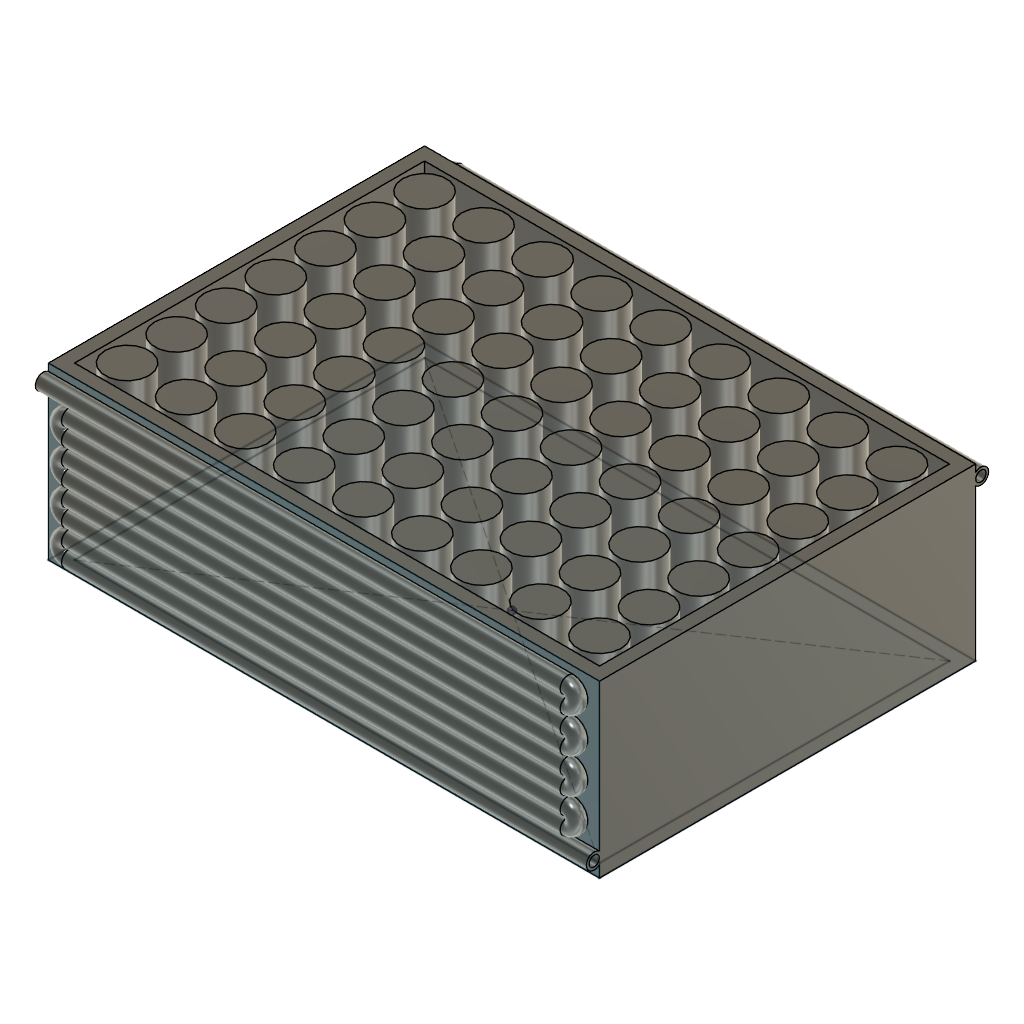
BATTERY_PACK_11 (Autodesk Fusion 360 design; units mm, degrees)
Autodesk Fusion 360 part; units mm, degrees
sketch "Sketch1" plane through (0, 0, 0) normal (0, 0, 1) x (1, 0, 0)
  line L0 (150, 100) -> (-150, 100)
  line L1 (-150, 100) -> (-150, -100)
  line L2 (-150, -100) -> (150, -100)
  line L3 (150, -100) -> (150, 100)
  line L4 (150, 100) -> (-150, -100) construction
  line L5 (-150, 100) -> (150, -100) construction
  line L6 (-157.5, -107.5) -> (157.5, -107.5)
  line L7 (157.5, -107.5) -> (157.5, 107.5)
  line L8 (157.5, 107.5) -> (-157.5, 107.5)
  line L9 (-157.5, 107.5) -> (-157.5, -107.5)
  dimension "d1" = 300
  dimension "d2" = 200
  dimension "d3" = 7.5
  constraint horizontal L0
  constraint perpendicular L0 L1
  constraint parallel L0 L2
  constraint parallel L1 L3
  constraint coincident L4 origin
  constraint coincident L5 origin
  measures "d1" distance of L1.end L2.end
  measures "d2" distance of L0.end L1.end
extrude "Extrude1" add sketch "Sketch1" along normal blind 7.5 contours L0 L1 L2 L3
extrude "Extrude2" add sketch "Sketch1" along normal blind 97.5
sketch "Sketch2" plane through (0, 0, 7.5) normal (0, 0, 1) x (-1, 0, 0)
  line L0 (-150, 100) -> (-150, -100)
  line L1 (-150, -100) -> (150, -100)
  line L2 (150, -100) -> (150, 100)
  line L3 (150, 100) -> (-150, 100)
  circle A0 centre (0, 0) radius 12.5
  circle A1 centre (33.75, 0) radius 12.5
  circle A2 centre (67.5, 0) radius 12.5
  circle A3 centre (101.25, 0) radius 12.5
  circle A4 centre (135, 0) radius 12.5
  circle A5 centre (0, 28.3333) radius 12.5
  circle A6 centre (33.75, 28.3333) radius 12.5
  circle A7 centre (67.5, 28.3333) radius 12.5
  circle A8 centre (101.25, 28.3333) radius 12.5
  circle A9 centre (135, 28.3333) radius 12.5
  circle A10 centre (0, 56.6667) radius 12.5
  circle A11 centre (33.75, 56.6667) radius 12.5
  circle A12 centre (67.5, 56.6667) radius 12.5
  circle A13 centre (101.25, 56.6667) radius 12.5
  circle A14 centre (135, 56.6667) radius 12.5
  circle A15 centre (0, 85) radius 12.5
  circle A16 centre (33.75, 85) radius 12.5
  circle A17 centre (67.5, 85) radius 12.5
  circle A18 centre (101.25, 85) radius 12.5
  circle A19 centre (135, 85) radius 12.5
  circle A20 centre (33.75, 0) radius 12.5
  circle A21 centre (67.5, 0) radius 12.5
  circle A22 centre (101.25, 0) radius 12.5
  circle A23 centre (135, 0) radius 12.5
  circle A24 centre (0, -28.3333) radius 12.5
  circle A25 centre (33.75, -28.3333) radius 12.5
  circle A26 centre (67.5, -28.3333) radius 12.5
  circle A27 centre (101.25, -28.3333) radius 12.5
  circle A28 centre (135, -28.3333) radius 12.5
  circle A29 centre (0, -56.6667) radius 12.5
  circle A30 centre (33.75, -56.6667) radius 12.5
  circle A31 centre (67.5, -56.6667) radius 12.5
  circle A32 centre (101.25, -56.6667) radius 12.5
  circle A33 centre (135, -56.6667) radius 12.5
  circle A34 centre (0, -85) radius 12.5
  circle A35 centre (33.75, -85) radius 12.5
  circle A36 centre (67.5, -85) radius 12.5
  circle A37 centre (101.25, -85) radius 12.5
  circle A38 centre (135, -85) radius 12.5
  circle A39 centre (-33.75, 0) radius 12.5
  circle A40 centre (-67.5, 0) radius 12.5
  circle A41 centre (-101.25, 0) radius 12.5
  circle A42 centre (-135, 0) radius 12.5
  circle A43 centre (0, -28.3333) radius 12.5
  circle A44 centre (-33.75, -28.3333) radius 12.5
  circle A45 centre (-67.5, -28.3333) radius 12.5
  circle A46 centre (-101.25, -28.3333) radius 12.5
  circle A47 centre (-135, -28.3333) radius 12.5
  circle A48 centre (0, -56.6667) radius 12.5
  circle A49 centre (-33.75, -56.6667) radius 12.5
  circle A50 centre (-67.5, -56.6667) radius 12.5
  circle A51 centre (-101.25, -56.6667) radius 12.5
  circle A52 centre (-135, -56.6667) radius 12.5
  circle A53 centre (0, -85) radius 12.5
  circle A54 centre (-33.75, -85) radius 12.5
  circle A55 centre (-67.5, -85) radius 12.5
  circle A56 centre (-101.25, -85) radius 12.5
  circle A57 centre (-135, -85) radius 12.5
  circle A58 centre (-33.75, 0) radius 12.5
  circle A59 centre (-67.5, 0) radius 12.5
  circle A60 centre (-101.25, 0) radius 12.5
  circle A61 centre (-135, 0) radius 12.5
  circle A62 centre (0, 28.3333) radius 12.5
  circle A63 centre (-33.75, 28.3333) radius 12.5
  circle A64 centre (-67.5, 28.3333) radius 12.5
  circle A65 centre (-101.25, 28.3333) radius 12.5
  circle A66 centre (-135, 28.3333) radius 12.5
  circle A67 centre (0, 56.6667) radius 12.5
  circle A68 centre (-33.75, 56.6667) radius 12.5
  circle A69 centre (-67.5, 56.6667) radius 12.5
  circle A70 centre (-101.25, 56.6667) radius 12.5
  circle A71 centre (-135, 56.6667) radius 12.5
  circle A72 centre (0, 85) radius 12.5
  circle A73 centre (-33.75, 85) radius 12.5
  circle A74 centre (-67.5, 85) radius 12.5
  circle A75 centre (-101.25, 85) radius 12.5
  circle A76 centre (-135, 85) radius 12.5
  dimension "d8" = 25
  dimension "d11" = 135
  dimension "d12" = 85
  dimension "d15" = 135
  dimension "d16" = -85
  dimension "d19" = -135
  dimension "d20" = -85
  dimension "d23" = -135
  dimension "d24" = 85
  constraint coincident A0.centre origin
  measures "d8" diameter of A0
extrude "Extrude3" add sketch "Sketch2" along normal blind 90 contours A0 | A1 A20 | A2 A21 | A3 A22 | A4 A23 | A5 A62 | A6 | A7 | A8 | A9 | A10 A67 | A11 | A12 | A13 | A14 | A15 A72 | A16 | A17 | A18 | A19 | A24 A43 | A25 | A26 | A27 | A28 | A29 A48 | A30 | A31 | A32 | A33 | A34 A53 | A35 | A36 | A37 | A38 | A39 A58 | A40 A59 | A41 A60 | A42 A61 | A44 | A45 | A46 | A47 | A49 | A50 | A51 | A52 | A54 | A55 | A56 | A57 | A63 | A64 | A65 | A66 | A68 | A69 | A70 | A71 | A73 | A74 | A75 | A76
ref_plane "WorkPlane1" through (0, -110.5, 48.75) normal (0, -1, 0) x (1, 0, 0)
sketch "Sketch3" plane through (0, -110.5, 0) normal (0, -1, 0) x (-1, 0, 0)
  line L0 (-157.5, -97.5) -> (-150, -97.5)
  line L1 (157.5, -90) -> (-142.5, -90)
  arc A0 (-142.5, -80) -> (-142.5, -90) centre (-142.5, -85) ccw
  line L2 (-142.5, -80) -> (142.5, -80)
  arc A1 (142.5, -80) -> (142.5, -70) centre (142.5, -75) ccw
  line L3 (142.5, -70) -> (-142.5, -70)
  arc A2 (-142.5, -60) -> (-142.5, -70) centre (-142.5, -65) ccw
  line L4 (-142.5, -60) -> (142.5, -60)
  arc A3 (142.5, -60) -> (142.5, -50) centre (142.5, -55) ccw
  line L5 (142.5, -50) -> (-142.5, -50)
  arc A4 (-142.5, -40) -> (-142.5, -50) centre (-142.5, -45) ccw
  line L6 (-142.5, -40) -> (142.5, -40)
  arc A5 (142.5, -40) -> (142.5, -30) centre (142.5, -35) ccw
  line L7 (142.5, -30) -> (-142.5, -30)
  arc A6 (-142.5, -20) -> (-142.5, -30) centre (-142.5, -25) ccw
  line L8 (-142.5, -20) -> (142.5, -20)
  arc A7 (142.5, -20) -> (142.5, -10) centre (142.5, -15) ccw
  line L9 (142.5, -10) -> (-157.5, -10)
  line L10 (142.5, -10) -> (442.4801, -10) construction
  line L11 (-157.5, 0) -> (-157.5, -97.5)
  line L12 (157.5, 0) -> (157.5, -97.5)
  line L13 (157.5, -97.5) -> (-157.5, -97.5)
  dimension "d33" = 7.5
  dimension "d34" = 300
  dimension "d35" = 285
  dimension "d36" = 180
  dimension "d37" = 5
  dimension "d38" = 5
  dimension "d39" = 5
  dimension "d40" = 5
  dimension "d41" = 5
  dimension "d42" = 5
  dimension "d43" = 5
  dimension "d44" = 5
  dimension "d45" = 15
  dimension "d46" = 40
  dimension "d47" = 20
  dimension "d48" = 285
  dimension "d49" = 285
  dimension "d50" = 300
  dimension "d51" = 15
  dimension "d52" = 15
  dimension "d53" = 7.5
  dimension "d54" = 15
  dimension "d55" = 15
  dimension "d56" = 15
  dimension "d57" = 15
  constraint horizontal L0
  constraint tangent L1 A0
  constraint parallel L1 L2
  constraint tangent L2 A1
  constraint tangent A1 L3
  constraint tangent L3 A2
  constraint tangent A2 L4
  constraint parallel L3 L4
  constraint tangent L4 A3
  constraint tangent A3 L5
  constraint tangent L5 A4
  constraint tangent A4 L6
  constraint parallel L5 L6
  constraint tangent L6 A5
  constraint tangent A5 L7
  constraint parallel L6 L7
  constraint tangent L7 A6
  constraint tangent A6 L8
  constraint parallel L7 L8
  constraint tangent L8 A7
  constraint tangent A7 L10
  measures "d33" distance of L0.start L0.end
  measures "d34" distance of L1.start L1.end
  measures "d35" distance of A0.start L2.end
  measures "d36" angle of L9 L10
  measures "d37" radius of A1
  measures "d38" radius of A3
  measures "d39" radius of A5
  measures "d40" radius of A7
  measures "d41" radius of A0
  measures "d42" radius of A2
  measures "d43" radius of A4
  measures "d44" radius of A6
  measures "d45" distance of L1 A1.centre
  measures "d46" distance of L1 L5
  measures "d47" distance of A3.centre A5.centre
  measures "d48" distance of A1.end L3.end
  measures "d49" distance of A5.end L7.end
  measures "d50" distance of A7.end L9.end
  measures "d51" distance of A2.centre L11
  measures "d52" distance of A1.centre L12
  measures "d53" distance of L1 L13
  measures "d54" distance of A3.centre L12
  measures "d55" distance of A7.centre L12
  measures "d56" distance of A4.centre L11
  measures "d57" distance of A6.centre L9
sketch "Sketch4" plane through (0, -107.5, 0) normal (0, -1, 0) x (1, 0, 0)
  line L0 (-157.5, 0) -> (157.5, 0)
  line L1 (157.5, 0) -> (157.5, 97.5)
  line L2 (157.5, 97.5) -> (-157.5, 97.5)
  line L3 (-157.5, 97.5) -> (-157.5, 0)
pipe "Pipe1" add diameter 9 wall 1.55 path "Sketch3" along L1 A0 L2 A1 L3 A2 L4 A3 L5 A4 L6 A5 L7 A6 L8 A7 L9
ref_plane "WorkPlane2" through (0, 110.5, 48.75) normal (0, 1, 0) x (-1, 0, 0)
sketch "Sketch5" plane through (0, 110.5, 0) normal (0, 1, 0) x (1, 0, 0)
  line L0 (157.5, -90) -> (-142.5, -90)
  arc A0 (-142.5, -80) -> (-142.5, -90) centre (-142.5, -85) ccw
  line L1 (-142.5, -80) -> (142.5, -80)
  arc A1 (142.5, -80) -> (142.5, -70) centre (142.5, -75) ccw
  line L2 (142.5, -70) -> (-142.5, -70)
  arc A2 (-142.5, -60) -> (-142.5, -70) centre (-142.5, -65) ccw
  line L3 (-142.5, -60) -> (142.5, -60)
  arc A3 (142.5, -60) -> (142.5, -50) centre (142.5, -55) ccw
  line L4 (142.5, -50) -> (-142.5, -50)
  arc A4 (-142.5, -40) -> (-142.5, -50) centre (-142.5, -45) ccw
  line L5 (-142.5, -40) -> (142.5, -40)
  arc A5 (142.5, -40) -> (142.5, -30) centre (142.5, -35) ccw
  line L6 (142.5, -30) -> (-142.5, -30)
  arc A6 (-142.5, -20) -> (-142.5, -30) centre (-142.5, -25) ccw
  line L7 (-142.5, -20) -> (142.5, -20)
  arc A7 (142.5, -20) -> (142.5, -10) centre (142.5, -15) ccw
  line L8 (142.5, -10) -> (-157.5, -10)
  line L9 (157.5, -97.5) -> (-157.5, -97.5)
  line L10 (157.5, 0) -> (157.5, -97.5)
  dimension "d66" = 300
  dimension "d67" = 285
  dimension "d68" = 5
  dimension "d69" = 5
  dimension "d70" = 5
  dimension "d71" = 15
  dimension "d72" = 7.5
  dimension "d73" = 80
  dimension "d74" = 15
  dimension "d75" = 15
  dimension "d76" = 15
  dimension "d77" = 15
  dimension "d78" = 5
  dimension "d79" = 285
  dimension "d80" = 285
  dimension "d81" = 285
  constraint tangent L0 A0
  constraint tangent A0 L1
  constraint tangent L1 A1
  constraint tangent A1 L2
  constraint tangent L2 A2
  constraint tangent A2 L3
  constraint parallel L2 L3
  constraint tangent L3 A3
  constraint tangent A3 L4
  constraint parallel L3 L4
  constraint tangent L4 A4
  constraint tangent A4 L5
  constraint parallel L4 L5
  constraint tangent L5 A5
  constraint tangent A5 L6
  constraint parallel L5 L6
  constraint tangent L6 A6
  constraint tangent A6 L7
  constraint parallel L6 L7
  constraint tangent L7 A7
  constraint tangent A7 L8
  constraint equal A2 A4
  constraint equal A2 A6
  constraint equal A3 A5
  constraint equal A1 A7
  measures "d66" distance of L0.start L0.end
  measures "d67" distance of A0.start L1.end
  measures "d68" radius of A1
  measures "d69" radius of A0
  measures "d70" radius of A2
  measures "d71" distance of L0 A1.centre
  measures "d72" distance of L0 L9
  measures "d73" distance of L0 L8
  measures "d74" distance of A7.centre L10
  measures "d75" distance of A5.centre L10
  measures "d76" distance of A3.centre L10
  measures "d77" distance of A1.centre L10
  measures "d78" radius of A3
  measures "d79" distance of A1.end L2.end
  measures "d80" distance of A3.end L4.end
  measures "d81" distance of A6.start L7.end
pipe "Pipe2" add diameter 9 wall 1.55 path "Sketch5" along L0 A0 L1 A1 L2 A2 L3 A3 L4 A4 L5 A5 L6 A6 L7 A7 L8
